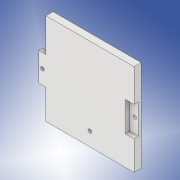
# Autodesk Inventor part: TA002
Saved by Autodesk Inventor 2017 SP1 (Build 210196100, 196)
## iProperties
Created: 2017-08-15
Part Number: TA002
Material: ABS Plastic
Document SubType Name: Modeling
Designer: Zach
Density: 1.06 g/cm^3
Appearance: CR White
Author: Zach
Autodesk Inventor part; units mm, degrees
ref_plane "YZ Plane" through (0, 0, 0) normal (1, 0, 0) x (0, 1, 0)
ref_plane "XZ Plane" through (0, 0, 0) normal (0, 1, 0) x (-1, 0, 0)
ref_plane "XY Plane" through (0, 0, 0) normal (0, 0, 1) x (1, 0, 0)
sketch "Sketch1" plane through (0, 0, 0) normal (0, 0, 1) x (1, 0, 0)
  line L0 (0, 0) -> (124, 0)
  line L1 (124, 0) -> (124, 129)
  line L2 (124, 129) -> (0, 129)
  line L3 (0, 129) -> (0, 0)
  circle A0 centre (62, 19.5) radius 2.5
  point P0 (62, 0)
  dimension "d0" = 124
  dimension "d1" = 129
  dimension "d2" = 5
  dimension "d3" = 19.5
  constraints: 8 end point, 2 parallel, 1 centre point, 1 horizontal, 1 midpoint, 1 perpendicular, 1 vertical alignment
  measures "d0" distance of L2.end L1.end
  measures "d1" distance of L1.end L0.end
  measures "d2" diameter of A0
  measures "d3" distance from line of L0 A0.centre
extrude "Extrusion1" add sketch "Sketch1" along normal blind 10
sketch "Sketch2" plane through (0, 0, 10) normal (0, 0, 1) x (1, 0, 0)
  line L0 (0, 82) -> (-10, 82)
  line L1 (-10, 82) -> (-10, 42)
  line L2 (-10, 42) -> (0, 42)
  line L3 (0, 42) -> (0, 82)
  circle A0 centre (-5, 62) radius 2.5
  line L4 (0, 124) -> (0, 0)
  line L5 (0, 129) -> (0, 0) projected
  point P0 (-10, 62)
  point P1 (0, 62)
  point P2 (-5, 82)
  point P3 (0, 62)
  dimension "d8" = 10
  dimension "d9" = 40
  dimension "d10" = 5
  dimension "d27" = 124
  constraints: 10 end point, 3 horizontal alignment, 3 midpoint, 2 parallel, 1 centre point, 1 horizontal, 1 perpendicular, 1 point on line, 1 vertical, 1 vertical alignment
  measures "d8" distance of L2.end L1.end
  measures "d9" distance of L1.end L0.end
  measures "d10" diameter of A0
  measures "d27" distance of L4.start L4.end
extrude "Extrusion2" add sketch "Sketch2" against normal blind 5
sketch "Sketch3" plane through (0, 0, 10) normal (0, 0, 1) x (1, 0, 0)
  line L0 (124, 41) -> (112, 41)
  line L1 (112, 41) -> (112, 83)
  line L2 (112, 83) -> (124, 83)
  line L3 (124, 83) -> (124, 41)
  line L4 (124, 0) -> (124, 129) projected
  line L5 (124, 124) -> (124, 0)
  point P0 (0, 0)
  point P1 (112, 62)
  point P2 (124, 62)
  point P3 (124, 62)
  dimension "d13" = 12
  dimension "d14" = 42
  dimension "d28" = 124
  constraints: 10 end point, 2 horizontal alignment, 2 midpoint, 2 parallel, 1 collinear, 1 horizontal, 1 perpendicular, 1 point on line
  measures "d13" distance of L1.end L2.end
  measures "d14" distance of L0.end L1.end
  measures "d28" distance of L5.start L4.start
extrude "Extrusion3" cut sketch "Sketch3" against normal blind 6
sketch "Sketch4" plane through (0, 0, 4) normal (0, 0, 1) x (1, 0, 0)
  line L0 (124, 41) -> (112, 41) construction
  line L1 (124, 83) -> (124, 41) construction
  line L2 (112, 83) -> (124, 83) construction
  line L3 (112, 41) -> (112, 83) construction
  circle A0 centre (119, 62) radius 2.5
  point P0 (0, 0)
  point P1 (124, 62)
  point P2 (118, 41)
  dimension "d17" = 5
  dimension "d29" = 5
  constraints: 2 midpoint, 1 centre point, 1 horizontal alignment
  measures "d17" diameter of A0
  measures "d29" distance of point (124, 62) A0.centre
extrude "Extrusion4" cut sketch "Sketch4" against normal through all
body "Solid1"
